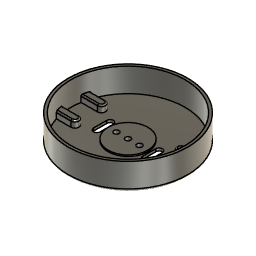
TRARM02_Link1A_R90x20 (Autodesk Fusion 360 design; units mm, degrees)
Autodesk Fusion 360 part; units mm, degrees
sketch "스케치1" plane through (0, 0, 0) normal (0, 0, 1) x (1, 0, 0)
  circle A0 centre (0, 0) radius 45
  dimension "d1" = 90
  constraint coincident A0.centre origin
  measures "d1" diameter of A0
extrude "돌출1" add sketch "스케치1" along normal blind 2
sketch "스케치2" plane through (0, 0, 2) normal (0, 0, 1) x (-1, 0, 0)
  circle A0 centre (0, 0) radius 45
  circle A1 centre (0, 0) radius 43
  dimension "d4" = 86
  dimension "d5" = 90
  constraint coincident A0.centre A1.centre
  measures "d4" diameter of A1
  measures "d5" diameter of A0
extrude "돌출2" add sketch "스케치2" along normal blind 18
fillet "필렛1" radius 2 1 edges at (-41.9547, -16.2727, 0)
sketch "스케치4" plane through (0, 0, 2) normal (0, 0, 1) x (-1, 0, 0)
  circle A0 centre (0, 0) radius 43
  line L0 (-30, -13) -> (-40.9878, -13)
  line L1 (-30, -7) -> (-42.4264, -7)
  line L2 (-30, 7) -> (-42.4264, 7)
  line L3 (-30, 13) -> (-40.9878, 13)
  line L4 (30, -13) -> (40.9878, -13)
  line L5 (30, -7) -> (42.4264, -7)
  line L6 (30, 7) -> (42.4264, 7)
  line L7 (30, 13) -> (40.9878, 13)
  arc A1 (30, 13) -> (30, 7) centre (30, 10) ccw
  arc A2 (30, -7) -> (30, -13) centre (30, -10) ccw
  arc A3 (-30, -13) -> (-30, -7) centre (-30, -10) ccw
  arc A4 (-30, 7) -> (-30, 13) centre (-30, 10) ccw
  dimension "d32" = 6
  dimension "d33" = 60
  dimension "d34" = 20
  dimension "d35" = 10
  dimension "d36" = 30
  dimension "d46" = 6
  dimension "d47" = 6
  constraint equal A2 A3
  constraint equal A1 A2
  constraint equal A1 A4
  constraint horizontal A2.centre A3.centre
  constraint horizontal A1.centre A4.centre
  constraint vertical A2.centre A1.centre
  constraint vertical A3.centre A4.centre
  constraint coincident A0 L0.end
  constraint coincident A0 L1.end
  constraint horizontal L0
  constraint horizontal L1
  constraint coincident A0 L2.end
  constraint coincident A0 L3.end
  constraint horizontal L2
  constraint horizontal L3
  constraint coincident A0 L4.end
  constraint coincident A0 L5.end
  constraint horizontal L4
  constraint horizontal L5
  constraint coincident A0 L6.end
  constraint coincident A0 L7.end
  constraint horizontal L6
  constraint horizontal L7
  constraint vertical L6.start L7.start
  constraint vertical L5.start L7.start
  constraint vertical L4.start L5.start
  constraint vertical L0.start L1.start
  constraint vertical L1.start L2.start
  constraint vertical L2.start L3.start
  measures "d32" diameter of A3
  measures "d33" distance of A2.centre A3.centre
  measures "d34" distance of A2.centre A1.centre
  measures "d35" vertical distance of A0.centre A1.centre
  measures "d36" horizontal distance of A0.centre A2.centre
  measures "d46" distance of L4 L5
  measures "d47" distance of L0 L1
extrude "돌출7" add sketch "스케치4" along normal blind 5 contours A0 L6 L7 A1 | A0 L4 L5 A2 | A0 L2 L3 A4 | A0 L0 L1 A3
sketch "스케치7" plane through (0, 0, 0) normal (0, 0, -1) x (1, 0, 0)
  arc A0 (-30, -13) -> (-30, -7) centre (-30, -10) ccw construction
  arc A1 (-30, 7) -> (-30, 13) centre (-30, 10) ccw construction
  arc A2 (30, 13) -> (30, 7) centre (30, 10) ccw construction
  arc A3 (30, -7) -> (30, -13) centre (30, -10) ccw construction
  circle A4 centre (-30, 10) radius 1.45
  circle A5 centre (-30, -10) radius 1.45
  circle A6 centre (30, -10) radius 1.45
  circle A7 centre (30, 10) radius 1.45
  dimension "d42" = 2.9
  constraint concentric A1 A4
  constraint concentric A0 A5
  constraint concentric A3 A6
  constraint concentric A2 A7
  constraint equal A6 A7
  constraint equal A5 A6
  constraint equal A4 A5
  measures "d42" diameter of A7
extrude "돌출8" cut sketch "스케치7" against normal blind 5
fillet "필렛2" radius 1 12 edges at (-35.4939, -13, 7) (-27, -10, 7) (-36.2132, -7, 7) (-36.2132, 7, 7) (-27, 10, 7) (-35.4939, 13, 7) (35.4939, 13, 7) (27, 10, 7) (36.2132, 7, 7) (36.2132, -7, 7) (27, -10, 7) (35.4939, -13, 7)
sketch "스케치9" plane through (0, 0, 2) normal (0, 0, 1) x (-1, 0, 0)
  circle A0 centre (0, 0) radius 15
  dimension "d50" = 30
  constraint coincident A0.centre origin
  measures "d50" diameter of A0
extrude "돌출9" add sketch "스케치9" along normal blind 1
sketch "스케치10" plane through (0, 0, 3) normal (0, 0, 1) x (-1, 0, 0)
  circle A0 centre (0, 0) radius 2
  circle A1 centre (-8.7, 0) radius 2
  circle A2 centre (8.7, 0) radius 2
  dimension "d53" = 8.7
  dimension "d54" = 8.7
  dimension "d55" = 4
  constraint coincident A0.centre origin
  constraint equal A0 A2
  constraint equal A1 A2
  constraint horizontal A0.centre A1.centre
  constraint horizontal A0.centre A2.centre
  measures "d53" distance of A0.centre A1.centre
  measures "d54" distance of A0.centre A2.centre
  measures "d55" diameter of A1
extrude "돌출10" cut sketch "스케치10" against normal blind 3
sketch "스케치11" plane through (0, 0, 0) normal (0, 0, -1) x (1, 0, 0)
  line L0 (21, 5) -> (21, -5)
  line L1 (16, -5) -> (16, 5)
  line L2 (-16, 5) -> (-16, -5)
  line L3 (-21, -5) -> (-21, 5)
  arc A0 (-16, 5) -> (-21, 5) centre (-18.5, 5) ccw
  arc A1 (-21, -5) -> (-16, -5) centre (-18.5, -5) ccw
  arc A2 (16, -5) -> (21, -5) centre (18.5, -5) ccw
  arc A3 (21, 5) -> (16, 5) centre (18.5, 5) ccw
  dimension "d58" = 5
  dimension "d60" = 10
  dimension "d61" = 16
  dimension "d62" = 5
  dimension "d63" = 16
  dimension "d64" = 2.5
  dimension "d65" = 5
  constraint vertical L0
  constraint vertical L1
  constraint vertical L2
  constraint vertical L3
  constraint equal L0 L2
  constraint horizontal L1.start L2.end
  constraint equal A2 A3
  constraint equal A0 A1
  constraint equal A0 A2
  constraint horizontal L3.end L2.start
  constraint horizontal L1.end L3.end
  constraint horizontal L1.end L0.start
  constraint equal L2 L3
  measures "d58" distance of L0.end L1.start
  measures "d60" distance of L0.start L0.end
  measures "d61" horizontal distance of origin L1.start
  measures "d62" vertical distance of origin L1.start
  measures "d63" horizontal distance of origin L2.end
  measures "d64" radius of A2
  measures "d65" distance of L2 L3
extrude "돌출11" cut sketch "스케치11" against normal blind 2
